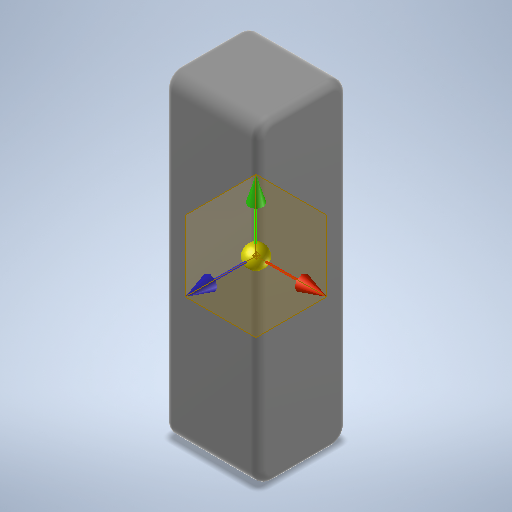
# Autodesk Inventor part: OVONIC 6S LiPo Battery
Saved by Autodesk Inventor 2026.2 (Build 302298010, 298A)
## iProperties
Created: 2026-03-12
Part Number: OVONIC 6S LiPo Battery
Material: PAEK Plastic
Document SubType Name: Modeling
Designer: tngzj
Density: 2.16665 g/cm^3
Appearance: Smooth - Dark Gray
Mass: 680 g
Surface Area: 303.039 cm^2
Volume: 313.849 cm^3
Author: tngzj
Autodesk Inventor part; units mm, degrees
ref_plane "YZ Plane" through (0, 0, 0) normal (1, 0, 0) x (0, 1, 0)
ref_plane "XZ Plane" through (0, 0, 0) normal (0, 1, 0) x (-1, 0, 0)
ref_plane "XY Plane" through (0, 0, 0) normal (0, 0, 1) x (1, 0, 0)
sketch "Sketch1" plane through (0, 0, 0) normal (0, 1, 0) x (-1, 0, 0)
  line L0 (-23.241, 21.971) -> (23.241, 21.971)
  line L1 (23.241, 21.971) -> (23.241, -21.971)
  line L2 (23.241, -21.971) -> (-23.241, -21.971)
  line L3 (-23.241, -21.971) -> (-23.241, 21.971)
  line L4 (-23.241, 21.971) -> (23.241, -21.971) construction
  line L5 (23.241, 21.971) -> (-23.241, -21.971) construction
  point P0 (0, 0)
  dimension "d0" = 46.482
  dimension "d1" = 43.942
  constraints: 12 end point, 2 midpoint, 2 parallel, 1 horizontal, 1 perpendicular
  measures "d0" distance of L0.start L0.end
  measures "d1" distance of L2.end L0.start
extrude "Extrusion1" add sketch "Sketch1" along normal blind 155.956
fillet "Fillet1" radius 7.62 4 edges at (0, 155.956, -21.971) (0, 155.956, 21.971) (0, 0, -21.971) (0, 0, 21.971)
fillet "Fillet2" radius 3.81 16 edges at (23.241, 153.7242, 19.7392) (23.241, 155.956, 0) (23.241, 153.7242, -19.7392) (23.241, 77.978, -21.971) (23.241, 2.2318, -19.7392) (23.241, 0, 0) (23.241, 2.2318, 19.7392) (23.241, 77.978, 21.971) (-23.241, 153.7242, 19.7392) (-23.241, 155.956, 0) (-23.241, 153.7242, -19.7392) (-23.241, 77.978, -21.971) (-23.241, 2.2318, -19.7392) (-23.241, 0, 0) (-23.241, 2.2318, 19.7392) (-23.241, 77.978, 21.971)
body "Solid1"
